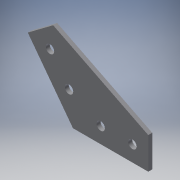
# Autodesk Inventor part: angle gusset plate
Saved by Autodesk Inventor 2016 (Build 200138000, 138)
## iProperties
Created: 2016-02-04
Part Number: angle gusset plate
Material: Generic
Document SubType Name: Modeling
Designer: gus
Density: 1 g/cm^3
Appearance: Default
Author: gus
Autodesk Inventor part; units mm, degrees
ref_plane "YZ Plane" through (0, 0, 0) normal (1, 0, 0) x (0, 1, 0)
ref_plane "XZ Plane" through (0, 0, 0) normal (0, 1, 0) x (-1, 0, 0)
ref_plane "XY Plane" through (0, 0, 0) normal (0, 0, 1) x (1, 0, 0)
sketch "Sketch1" plane through (0, 0, 0) normal (0, 0, 1) x (1, 0, 0)
  line L0 (0, 0) -> (73.025, 0)
  line L1 (73.025, 0) -> (73.025, 25.4)
  line L2 (73.025, 25.4) -> (-25.4001, 76.2)
  line L3 (-25.4001, 76.2) -> (-45.7201, 60.9599)
  line L4 (-45.7201, 60.9599) -> (0, 0)
  circle A0 centre (60.325, 12.7) radius 3.3734
  circle A1 centre (34.925, 12.7) radius 3.3734
  circle A2 centre (2.54, 17.78) radius 3.3734
  circle A3 centre (-27.9401, 58.42) radius 3.3734
  line L5 (73.025, 12.7) -> (-9.525, 12.7) construction
  line L6 (-35.5601, 68.5799) -> (15.875, 0) construction
  line L7 (0, 0) -> (49.8292, 37.372) construction
  line L8 (20.32, 15.24) -> (12.7, 25.4) construction
  circle A4 centre (-12.7001, 38.1) radius 3.3734
  dimension "d0" = 73.025
  dimension "d1" = 25.4
  dimension "d2" = 25.4
  dimension "d3" = 76.2
  dimension "d4" = 126.87
  dimension "d5" = 6.7469
  dimension "d6" = 25.4
  dimension "d7" = 12.7
  dimension "d8" = 12.7
  dimension "d12" = 12.7
  dimension "d13" = 25.4
  dimension "d14" = 12.7
  dimension "d15" = 38.1
  constraints: 18 end point, 9 point on line, 5 centre point, 4 equal radius, 4 perpendicular, 2 midpoint, 1 horizontal, 1 parallel
  measures "d0" distance of L0.start L0.end
  measures "d1" distance of L0.end L1.end
  measures "d2" distance of L2.end L3.end
  measures "d3" distance of L3.end L0.start
  measures "d4" angle of L4 L0
  measures "d5" diameter of A0
  measures "d6" distance of A1.centre A0.centre
  measures "d7" distance from line of L1 A0.centre
  measures "d8" distance from line of L3 A3.centre
  measures "d12" distance from line of L7 A2.centre
  measures "d13" distance between parallel lines of L4 L8
  measures "d14" distance of L8.start L8.end
  measures "d15" distance from line of L3 A4.centre
extrude "Extrusion1" add sketch "Sketch1" along normal blind 3.175 contours L4 L3 L2 L1 L0 | A4
body "Solid1"
